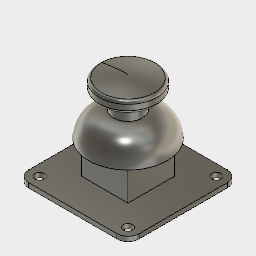
512 Thumb Joystick (Autodesk Fusion 360 design; units mm, degrees)
Autodesk Fusion 360 part; units mm, degrees
note: some values were not read from the file. Set by a fixed rule: which sketch regions a step uses.
sketch "Sketch1" plane through (0, 0, 0) normal (0, 0, 1) x (1, 0, 0)
  circle A0 centre (3.81, 34.29) radius 1.6
  arc A1 (38.1, 34.29) -> (34.29, 38.1) centre (34.29, 34.29) ccw
  arc A2 (3.81, 38.1) -> (0, 34.29) centre (3.81, 34.29) ccw
  circle A3 centre (34.29, 34.29) radius 1.6
  line L0 (34.29, 38.1) -> (3.81, 38.1)
  arc A4 (34.29, 0) -> (38.1, 3.81) centre (34.29, 3.81) ccw
  circle A5 centre (3.81, 3.81) radius 1.6
  circle A6 centre (34.29, 3.81) radius 1.6
  line L1 (3.81, 0) -> (34.29, 0)
  arc A7 (0, 3.81) -> (3.81, 0) centre (3.81, 3.81) ccw
  line L2 (38.1, 3.81) -> (38.1, 34.29)
  line L3 (0, 34.29) -> (0, 3.81)
  dimension "d1" = 30.48
  dimension "d2" = 30.48
  measures "d1" distance of A0.centre A1.centre
  measures "d2" distance of A1.centre A4.centre
extrude "Extrude1" add sketch "Sketch1" along normal blind 1.6 makes body 1
sketch "Sketch2" plane through (0, 0, 1.6) normal (0, 0, 1) x (-1, 0, 0)
  circle A0 centre (-34.29, -34.29) radius 1.6
  circle A1 centre (-3.81, -3.81) radius 1.6
  circle A2 centre (-34.29, -3.81) radius 1.6
  circle A3 centre (-3.81, -34.29) radius 1.6
  line L0 (0, -34.29) -> (0, -3.81)
  arc A4 (0, -3.81) -> (-3.81, 0) centre (-3.81, -3.81) ccw
  line L1 (-3.81, 0) -> (-34.29, 0)
  arc A5 (-34.29, 0) -> (-38.1, -3.81) centre (-34.29, -3.81) ccw
  line L2 (-38.1, -3.81) -> (-38.1, -34.29)
  arc A6 (-38.1, -34.29) -> (-34.29, -38.1) centre (-34.29, -34.29) ccw
  line L3 (-34.29, -38.1) -> (-3.81, -38.1)
  arc A7 (-3.81, -38.1) -> (0, -34.29) centre (-3.81, -34.29) ccw
  line L4 (0, -19.05) -> (-38.1, -19.05) construction
  line L5 (-19.05, -38.1) -> (-19.05, 0) construction
  line L6 (-27.05, -11.05) -> (-11.05, -11.05)
  line L7 (-11.05, -11.05) -> (-11.05, -27.05)
  line L8 (-11.05, -27.05) -> (-27.05, -27.05)
  line L9 (-27.05, -27.05) -> (-27.05, -11.05)
  line L10 (-27.05, -11.05) -> (-11.05, -27.05) construction
  line L11 (-11.05, -11.05) -> (-27.05, -27.05) construction
  circle A8 centre (-19.05, -19.05) radius 13.5
  point P0 (-19.05, -19.05)
  dimension "d5" = 16
  dimension "d6" = 16
  dimension "d7" = 27
  measures "d5" distance of L7.end L8.end
  measures "d6" distance of L6.end L7.end
  measures "d7" diameter of A8
extrude "Extrude2" add sketch "Sketch2" along normal blind 11.4 separate body contours L6 L7 L8 L9 makes body 2
extrude "Extrude3" add sketch "Sketch2" along normal blind 8.5 from surface at 11.4 contours L6 L7 L8 L9 | A8 bodies 2
fillet "Fillet1" radius 8.5 1 edges at (31.6364, 23.9318, 21.5) on bodies 2
extrude "Extrude4" add 1 faces at (16.1101, 20.07, 21.5) along direction (0, 0, 1) blind 4.5 on bodies 2 bodies 2
sketch "Sketch3" plane through (0, 0, 26) normal (0, 0, 1) x (-1, 0, 0)
  circle A0 centre (-19.05, -19.05) radius 5
  circle A1 centre (-19.05, -19.05) radius 9.9
  dimension "d16" = 19.8
  measures "d16" diameter of A1
extrude "Extrude5" add sketch "Sketch3" along normal blind 6 separate body contours A0 | A1 makes body 3
sketch "Sketch4" plane through (0, 0, 0) normal (0, 1, 0) x (1, 0, 0)
  line L0 (24.05, -21.5) -> (14.05, -21.5)
  line L1 (9.15, -32) -> (28.95, -32)
  line L2 (9.15, -26) -> (28.95, -26)
  line L3 (14.05, -26) -> (9.8664, -27.1996)
  line L4 (9.142, -28.1609) -> (9.142, -30.0648)
  line L5 (19.05, -26) -> (19.05, -32)
  spline S0 degree 5 poles (9.9755, -31.0509) (10.1966, -31.0882) (10.8062, -31.1897) (11.8064, -31.35) (13.2013, -31.5579) (15.0011, -31.7875) (16.5987, -31.9299) (17.8159, -31.9872) (18.637, -32) (19.05, -32) knots 0.086035 0.086035 0.086035 0.086035 0.086035 0.086035 0.2 0.4 0.6 0.8 1 1 1 1 1 1
  line L6 (18, -32) -> (20.1, -32)
  arc A0 (9.142, -30.0648) -> (9.9755, -31.0509) centre (10.142, -30.0648) ccw
  line L7 (14.05, -26) -> (24.05, -26)
  arc A1 (9.8664, -27.1996) -> (9.142, -28.1609) centre (10.142, -28.1609) ccw
  point P0 (9.142, -27.4073)
  point P1 (9.142, -29.9073)
  dimension "d19" = 16
  dimension "d20" = 2.5
  dimension "d21" = 1
  dimension "d23" = 1
  measures "d19" angle of L2 L3
  measures "d20" distance of P0 P1
  measures "d21" radius of A0
  measures "d23" radius of A1
revolve "Revolve1" add sketch "Sketch4" angle 360 about axis through (19.05, 0, 26) along (0, 0, 1) separate body makes body 4
move_body "Move1" bodies 4 to x (1, 0, 0) y (0, 1, 0) z (0, 0, 1) at (0, 19.05, 0)
hidden bodies 3
